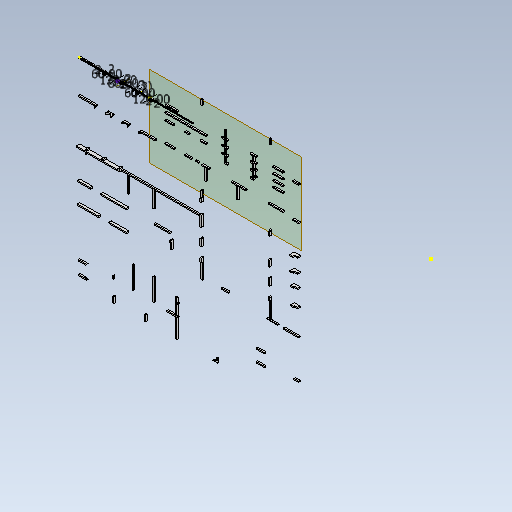
# Autodesk Inventor part: SPRUEs
Saved by Autodesk Inventor 2023 (Build 270158030, 158C)
## iProperties
Created: 2024-12-30
Part Number: SPRUEs
Material: Generic
Document SubType Name: Modeling
Designer: Imogen Heard
Density: 1 g/cm^3
Appearance: Default
Author: Imogen Heard
Autodesk Inventor part; units mm, degrees
(part 1 of 2)
ref_plane "YZ Plane" through (0, 0, 0) normal (1, 0, 0) x (0, 1, 0)
ref_plane "XZ Plane" through (0, 0, 0) normal (0, 1, 0) x (-1, 0, 0)
ref_plane "XY Plane" through (0, 0, 0) normal (0, 0, 1) x (1, 0, 0)
sketch "Sketch1" plane through (0, 0, 0) normal (0, 0, 1) x (1, 0, 0)
  arc A0 (-355.3721, 16.6489) -> (-360.3721, 11.6489) centre (-355.3721, 11.6489) ccw projected
  line L0 (-360.3721, 11.6489) -> (-360.3721, -208.3511) projected
  arc A1 (-360.3721, -208.3511) -> (-355.3721, -213.3511) centre (-355.3721, -208.3511) ccw projected
  line L1 (-355.3721, -213.3511) -> (-135.3721, -213.3511) projected
  arc A2 (-135.3721, -213.3511) -> (-130.3721, -208.3511) centre (-135.3721, -208.3511) ccw projected
  line L2 (-130.3721, -208.3511) -> (-130.3721, 11.6489) projected
  arc A3 (-130.3721, 11.6489) -> (-135.3721, 16.6489) centre (-135.3721, 11.6489) ccw projected
  line L3 (-135.3721, 16.6489) -> (-355.3721, 16.6489) projected
  line L4 (-357.3721, -205.3511) -> (-357.3721, 8.6489) projected
  arc A4 (-352.3721, 13.6489) -> (-357.3721, 8.6489) centre (-352.3721, 8.6489) ccw projected
  line L5 (-352.3721, 13.6489) -> (-138.3721, 13.6489) projected
  arc A5 (-133.3721, 8.6489) -> (-138.3721, 13.6489) centre (-138.3721, 8.6489) ccw projected
  line L6 (-133.3721, 8.6489) -> (-133.3721, -205.3511) projected
  arc A6 (-138.3721, -210.3511) -> (-133.3721, -205.3511) centre (-138.3721, -205.3511) ccw projected
  line L7 (-138.3721, -210.3511) -> (-352.3721, -210.3511) projected
  arc A7 (-357.3721, -205.3511) -> (-352.3721, -210.3511) centre (-352.3721, -205.3511) ccw projected
  line L8 (-139.3721, -46.3511) -> (-139.3721, -11.3511) projected
  arc A8 (-139.3721, -11.3511) -> (-159.3721, 8.6489) centre (-159.3721, -11.3511) ccw projected
  arc A9 (-159.3721, -66.3511) -> (-139.3721, -46.3511) centre (-159.3721, -46.3511) ccw projected
  line L9 (-259.3721, -66.3511) -> (-159.3721, -66.3511) projected
  arc A10 (-279.3721, -46.3511) -> (-259.3721, -66.3511) centre (-259.3721, -46.3511) ccw projected
  line L10 (-279.3721, -11.3511) -> (-279.3721, -46.3511) projected
  arc A11 (-259.3721, 8.6489) -> (-279.3721, -11.3511) centre (-259.3721, -11.3511) ccw projected
  line L11 (-159.3721, 8.6489) -> (-259.3721, 8.6489) projected
  line L12 (-139.3721, -92.3511) -> (-139.3721, -72.8511) projected
  line L13 (-264.3721, -80.2511) -> (-264.3721, -77.8511) projected
  line L14 (-264.3721, -85.8511) -> (-264.3721, -83.4511) projected
  line L15 (-286.3721, 7.6489) -> (-290.1379, 7.6489) projected
  line L16 (-284.3721, -19.3481) -> (-284.3721, 5.6489) projected
  line L17 (-295.1379, 2.6489) -> (-295.1379, -19.3481) projected
  line L18 (-309.4963, -82.3511) -> (-284.3721, -19.3481) projected
  line L19 (-320.2621, -82.3511) -> (-295.1379, -19.3481) projected
  line L20 (-310.5821, -87.3511) -> (-318.1621, -87.3511) projected
  line L21 (-309.4963, -82.3511) -> (-320.2621, -82.3511) projected
  line L22 (-290.1379, 7.6489) -> (-286.3721, 7.6489) projected
  line L23 (-311.9037, -19.3481) -> (-311.9037, 2.6489) projected
  line L24 (-301.1379, -19.3481) -> (-301.1379, 5.6489) projected
  line L25 (-303.1379, 7.6489) -> (-306.9037, 7.6489) projected
  line L26 (-334.9279, -87.3511) -> (-327.3479, -87.3511) projected
  line L27 (-337.0279, -82.3511) -> (-311.9037, -19.3481) projected
  line L28 (-326.2621, -82.3511) -> (-301.1379, -19.3481) projected
  line L29 (-328.6695, 2.6489) -> (-328.6695, -19.3481) projected
  line L30 (-317.9037, 5.6489) -> (-317.9037, -19.3481) projected
  line L31 (-323.6695, 7.6489) -> (-319.9037, 7.6489) projected
  line L32 (-323.6695, 7.6489) -> (-319.9037, 7.6489) projected
  line L33 (-317.9037, -19.3481) -> (-343.0279, -82.3511) projected
  line L34 (-344.1137, -87.3511) -> (-351.6937, -87.3511) projected
  line L35 (-343.0279, -82.3511) -> (-353.7937, -82.3511) projected
  line L36 (-326.2621, -82.3511) -> (-337.0279, -82.3511) projected
  line L37 (-328.6695, -19.3481) -> (-353.7937, -82.3511) projected
  line L38 (-328.6695, -159.3541) -> (-353.7937, -96.3511) projected
  line L39 (-351.6937, -91.3511) -> (-344.1137, -91.3511) projected
  line L40 (-357.3721, -205.3511) -> (-357.3721, 8.6489) projected
  line L41 (-344.3835, -98.3511) -> (-350.843, -98.3511) projected
  line L42 (-353.7937, -96.3511) -> (-343.0279, -96.3511) projected
  line L43 (-343.0279, -96.3511) -> (-317.9037, -159.3541) projected
  line L44 (-344.3835, -80.3511) -> (-350.843, -80.3511) projected
  line L45 (-334.0772, -80.3511) -> (-327.6177, -80.3511) projected
  line L46 (-310.8519, -80.3511) -> (-317.3114, -80.3511) projected
  line L47 (-328.6695, -181.3511) -> (-328.6695, -159.3541) projected
  line L48 (-317.9037, -184.3511) -> (-317.9037, -159.3541) projected
  line L49 (-319.9037, -186.3511) -> (-323.6695, -186.3511) projected
  line L50 (-348.3721, -189.3511) -> (-350.1721, -191.1511) projected
  line L51 (-350.1721, -202.5511) -> (-348.3721, -204.3511) projected
  line L52 (-348.3721, -204.3511) -> (-315.3721, -204.3511) projected
  line L53 (-315.3721, -189.3511) -> (-348.3721, -189.3511) projected
  line L54 (-305.3721, -189.3511) -> (-267.3721, -189.3511) projected
  line L55 (-305.3721, -204.3511) -> (-267.3721, -204.3511) projected
  line L56 (-267.3721, -204.3511) -> (-267.3721, -202.3511) projected
  line L57 (-267.3721, -191.3511) -> (-267.3721, -189.3511) projected
  line L58 (-256.3721, -188.8511) -> (-256.3721, -190.8511) projected
  line L59 (-255.3721, -188.8511) -> (-256.3721, -188.8511) projected
  line L60 (-256.3721, -178.8511) -> (-256.3721, -176.8511) projected
  line L61 (-255.3721, -176.725) -> (-255.3721, -178.8511) projected
  line L62 (-177.3721, -187.8511) -> (-255.3721, -187.8511) projected
  line L63 (-255.3811, -191.985) -> (-220.3631, -196.7172) projected
  line L64 (-177.3631, -191.985) -> (-212.3811, -196.7172) projected
  line L65 (-217.8721, -206.3511) -> (-214.8721, -206.3511) projected
  line L66 (-176.3721, -190.8511) -> (-176.3721, -188.8511) projected
  line L67 (-176.3721, -176.8511) -> (-176.3721, -178.8511) projected
  line L68 (-212.3811, -170.985) -> (-177.3631, -175.7172) projected
  line L69 (-177.3721, -179.8511) -> (-255.3721, -179.8511) projected
  line L70 (-255.3811, -175.7172) -> (-220.3631, -170.985) projected
  line L71 (-217.8721, -161.3511) -> (-214.8721, -161.3511) projected
  line L72 (-168.1757, -199.4489) -> (-168.1757, -171.8085) projected
  line L73 (-139.3555, -200.6287) -> (-166.9959, -200.6287) projected
  line L74 (-138.1757, -171.8085) -> (-138.1757, -199.4489) projected
  line L75 (-166.9959, -170.6287) -> (-139.3555, -170.6287) projected
  spline S0 degree 3 poles (-166.3828, -172.4216) (-166.3184, -172.3571) (-166.2458, -172.3022) (-166.0818, -172.2096) (-165.9909, -172.1749) (-165.7801, -172.1268) (-165.6611, -172.1222) (-165.4156, -172.1541) (-165.2916, -172.1967) (-165.1278, -172.2899) (-165.0777, -172.3249) (-165.0079, -172.3837) (-164.9855, -172.4044) (-164.9474, -172.443) (-164.9314, -172.4605) (-164.8992, -172.498) (-164.8832, -172.5183) (-164.8443, -172.5717) (-164.8224, -172.6057) (-164.7512, -172.7333) (-164.7138, -172.8345) (-164.67, -173.0645) (-164.6692, -173.1941) (-164.7179, -173.4393) (-164.7617, -173.5526) (-164.8861, -173.7526) (-164.9616, -173.8378) (-165.1383, -173.9796) (-165.2367, -174.0339) (-165.449, -174.1095) (-165.5609, -174.1282) (-165.8051, -174.1293) (-165.9347, -174.103) (-166.1122, -174.0306) (-166.1684, -174.0012) (-166.2471, -173.95) (-166.2722, -173.9319) (-166.3151, -173.898) (-166.3332, -173.8826) (-166.3696, -173.8493) (-166.3878, -173.8313) (-166.4323, -173.7838) (-166.4576, -173.7534) (-166.5406, -173.6406) (-166.5883, -173.5503) (-166.6641, -173.3292) (-166.6831, -173.1946) (-166.6644, -172.9351) (-166.6331, -172.8127) (-166.5293, -172.5958) (-166.4637, -172.5025) (-166.3828, -172.4216) knots -0.679682 -0.679682 -0.679682 -0.679682 -0.652333 -0.652333 -0.622445 -0.622445 -0.584314 -0.584314 -0.540491 -0.540491 -0.519433 -0.519433 -0.508858 -0.508858 -0.50064 -0.50064 -0.491726 -0.491726 -0.477797 -0.477797 -0.44161 -0.44161 -0.400083 -0.400083 -0.362912 -0.362912 -0.328842 -0.328842 -0.294828 -0.294828 -0.25925 -0.25925 -0.215821 -0.215821 -0.194179 -0.194179 -0.183492 -0.183492 -0.175261 -0.175261 -0.166401 -0.166401 -0.152709 -0.152709 -0.117956 -0.117956 -0.073549 -0.073549 -0.034305 -0.034305 0 0 0 0 projected
  spline S1 degree 3 poles (-166.3828, -198.8358) (-166.4473, -198.7713) (-166.5022, -198.6988) (-166.5949, -198.5347) (-166.6295, -198.4439) (-166.6776, -198.2331) (-166.6822, -198.1141) (-166.6503, -197.8686) (-166.6078, -197.7446) (-166.5145, -197.5808) (-166.4795, -197.5307) (-166.4207, -197.4609) (-166.4, -197.4385) (-166.3614, -197.4004) (-166.344, -197.3844) (-166.3064, -197.3522) (-166.2862, -197.3362) (-166.2328, -197.2972) (-166.1987, -197.2754) (-166.0711, -197.2042) (-165.9699, -197.1668) (-165.7399, -197.123) (-165.6103, -197.1222) (-165.3651, -197.1709) (-165.2518, -197.2147) (-165.0518, -197.3391) (-164.9666, -197.4146) (-164.8248, -197.5913) (-164.7705, -197.6897) (-164.695, -197.902) (-164.6763, -198.0138) (-164.6751, -198.2581) (-164.7014, -198.3877) (-164.7738, -198.5652) (-164.8032, -198.6214) (-164.8544, -198.7) (-164.8725, -198.7252) (-164.9064, -198.7681) (-164.9219, -198.7862) (-164.9552, -198.8226) (-164.9731, -198.8408) (-165.0206, -198.8852) (-165.051, -198.9106) (-165.1638, -198.9936) (-165.2541, -199.0413) (-165.4752, -199.1171) (-165.6098, -199.136) (-165.8694, -199.1173) (-165.9917, -199.0861) (-166.2087, -198.9823) (-166.302, -198.9167) (-166.3828, -198.8358) knots -0.679682 -0.679682 -0.679682 -0.679682 -0.652333 -0.652333 -0.622445 -0.622445 -0.584314 -0.584314 -0.540491 -0.540491 -0.519433 -0.519433 -0.508858 -0.508858 -0.50064 -0.50064 -0.491726 -0.491726 -0.477797 -0.477797 -0.44161 -0.44161 -0.400083 -0.400083 -0.362912 -0.362912 -0.328842 -0.328842 -0.294828 -0.294828 -0.25925 -0.25925 -0.215821 -0.215821 -0.194179 -0.194179 -0.183492 -0.183492 -0.175261 -0.175261 -0.166401 -0.166401 -0.152709 -0.152709 -0.117956 -0.117956 -0.073549 -0.073549 -0.034305 -0.034305 0 0 0 0 projected
  spline S2 degree 3 poles (-139.9686, -198.8358) (-140.0331, -198.9003) (-140.1056, -198.9552) (-140.2697, -199.0478) (-140.3605, -199.0825) (-140.5713, -199.1306) (-140.6903, -199.1352) (-140.9359, -199.1033) (-141.0598, -199.0607) (-141.2237, -198.9675) (-141.2737, -198.9325) (-141.3435, -198.8737) (-141.3659, -198.853) (-141.404, -198.8144) (-141.42, -198.7969) (-141.4522, -198.7594) (-141.4682, -198.7391) (-141.5072, -198.6857) (-141.529, -198.6517) (-141.6003, -198.5241) (-141.6377, -198.4229) (-141.6815, -198.1929) (-141.6823, -198.0633) (-141.6335, -197.8181) (-141.5897, -197.7048) (-141.4653, -197.5048) (-141.3899, -197.4196) (-141.2131, -197.2778) (-141.1147, -197.2235) (-140.9024, -197.1479) (-140.7906, -197.1292) (-140.5463, -197.1281) (-140.4167, -197.1544) (-140.2392, -197.2268) (-140.183, -197.2562) (-140.1044, -197.3074) (-140.0792, -197.3255) (-140.0363, -197.3594) (-140.0182, -197.3749) (-139.9819, -197.4081) (-139.9637, -197.4261) (-139.9192, -197.4736) (-139.8939, -197.504) (-139.8108, -197.6168) (-139.7632, -197.7071) (-139.6873, -197.9282) (-139.6684, -198.0628) (-139.6871, -198.3223) (-139.7183, -198.4447) (-139.8222, -198.6616) (-139.8878, -198.7549) (-139.9686, -198.8358) knots -0.679682 -0.679682 -0.679682 -0.679682 -0.652333 -0.652333 -0.622445 -0.622445 -0.584314 -0.584314 -0.540491 -0.540491 -0.519433 -0.519433 -0.508858 -0.508858 -0.50064 -0.50064 -0.491726 -0.491726 -0.477797 -0.477797 -0.44161 -0.44161 -0.400083 -0.400083 -0.362912 -0.362912 -0.328842 -0.328842 -0.294828 -0.294828 -0.25925 -0.25925 -0.215821 -0.215821 -0.194179 -0.194179 -0.183492 -0.183492 -0.175261 -0.175261 -0.166401 -0.166401 -0.152709 -0.152709 -0.117956 -0.117956 -0.073549 -0.073549 -0.034305 -0.034305 0 0 0 0 projected
  spline S3 degree 3 poles (-139.9686, -172.4216) (-139.9041, -172.4861) (-139.8492, -172.5586) (-139.7566, -172.7227) (-139.722, -172.8135) (-139.6738, -173.0243) (-139.6692, -173.1433) (-139.7011, -173.3888) (-139.7437, -173.5128) (-139.837, -173.6766) (-139.8719, -173.7267) (-139.9308, -173.7965) (-139.9515, -173.8189) (-139.99, -173.857) (-140.0075, -173.873) (-140.0451, -173.9052) (-140.0653, -173.9212) (-140.1187, -173.9602) (-140.1528, -173.982) (-140.2803, -174.0532) (-140.3815, -174.0906) (-140.6115, -174.1344) (-140.7411, -174.1352) (-140.9864, -174.0865) (-141.0996, -174.0427) (-141.2996, -173.9183) (-141.3848, -173.8428) (-141.5266, -173.6661) (-141.5809, -173.5677) (-141.6565, -173.3554) (-141.6752, -173.2436) (-141.6764, -172.9993) (-141.65, -172.8697) (-141.5777, -172.6922) (-141.5482, -172.636) (-141.497, -172.5574) (-141.4789, -172.5322) (-141.445, -172.4893) (-141.4296, -172.4712) (-141.3963, -172.4348) (-141.3783, -172.4166) (-141.3309, -172.3722) (-141.3004, -172.3468) (-141.1876, -172.2638) (-141.0973, -172.2161) (-140.8762, -172.1403) (-140.7416, -172.1214) (-140.4821, -172.1401) (-140.3597, -172.1713) (-140.1428, -172.2751) (-140.0495, -172.3407) (-139.9686, -172.4216) knots -0.679682 -0.679682 -0.679682 -0.679682 -0.652333 -0.652333 -0.622445 -0.622445 -0.584314 -0.584314 -0.540491 -0.540491 -0.519433 -0.519433 -0.508858 -0.508858 -0.50064 -0.50064 -0.491726 -0.491726 -0.477797 -0.477797 -0.44161 -0.44161 -0.400083 -0.400083 -0.362912 -0.362912 -0.328842 -0.328842 -0.294828 -0.294828 -0.25925 -0.25925 -0.215821 -0.215821 -0.194179 -0.194179 -0.183492 -0.183492 -0.175261 -0.175261 -0.166401 -0.166401 -0.152709 -0.152709 -0.117956 -0.117956 -0.073549 -0.073549 -0.034305 -0.034305 0 0 0 0 projected
  circle A12 centre (-153.1757, -185.6287) radius 3 projected
  spline S4 degree 3 poles (-148.8989, -145.1578) (-148.8663, -145.2434) (-148.839, -145.3309) (-148.7526, -145.6882) (-148.7409, -145.9642) (-148.8289, -146.5268) (-148.9339, -146.8021) (-149.2681, -147.3464) (-149.5104, -147.5979) (-150.1323, -148.0483) (-150.5268, -148.2212) (-151.3838, -148.424) (-151.8499, -148.4418) (-152.6494, -148.3191) (-152.9891, -148.214) (-153.5655, -147.9256) (-153.8098, -147.7577) (-154.2292, -147.356) (-154.4037, -147.1255) (-154.6596, -146.6092) (-154.7368, -146.33) (-154.7716, -145.762) (-154.7323, -145.4845) (-154.5381, -144.9245) (-154.3742, -144.6555) (-153.9118, -144.1374) (-153.5973, -143.9109) (-152.9428, -143.5977) (-152.6093, -143.4993) (-151.9298, -143.4014) (-151.5828, -143.4016) (-150.877, -143.5041) (-150.5185, -143.6147) (-149.8769, -143.9427) (-149.5919, -144.1542) (-149.1611, -144.6332) (-149.0033, -144.8834) (-148.8989, -145.1578) knots -1.730763 -1.730763 -1.730763 -1.730763 -1.703218 -1.703218 -1.620235 -1.620235 -1.532045 -1.532045 -1.428588 -1.428588 -1.3023 -1.3023 -1.165882 -1.165882 -1.060948 -1.060948 -0.972967 -0.972967 -0.886826 -0.886826 -0.800067 -0.800067 -0.716091 -0.716091 -0.622376 -0.622376 -0.508288 -0.508288 -0.40586 -0.40586 -0.303624 -0.303624 -0.193192 -0.193192 -0.088285 -0.088285 0 0 0 0 projected
  arc A13 (-176.8395, -141.8511) -> (-181.3395, -141.8511) centre (-179.0895, -141.8511) ccw projected
  line L76 (-166.0395, -146.5637) -> (-166.0395, -145.5637) projected
  line L77 (-185.6895, -139.6011) -> (-185.6895, -140.8011) projected
  arc A14 (-184.6395, -141.8511) -> (-185.6895, -140.8011) centre (-185.6895, -141.8511) ccw projected
  line L78 (-184.6395, -141.8511) -> (-184.6395, -144.1637) projected
  arc A15 (-184.6395, -144.1637) -> (-180.1395, -144.1637) centre (-182.3895, -144.1637) ccw projected
  line L79 (-180.1395, -144.1637) -> (-180.1395, -141.8511) projected
  arc A16 (-178.0395, -141.8511) -> (-180.1395, -141.8511) centre (-179.0895, -141.8511) ccw projected
  line L80 (-178.0395, -141.8511) -> (-178.0395, -144.1637) projected
  arc A17 (-178.0395, -144.1637) -> (-173.0395, -144.1637) centre (-175.5395, -144.1637) ccw projected
  line L81 (-173.0395, -144.1637) -> (-173.0395, -141.8511) projected
  arc A18 (-170.4395, -141.8511) -> (-173.0395, -141.8511) centre (-171.7395, -141.8511) ccw projected
  line L82 (-170.4395, -141.8511) -> (-170.4395, -144.1637) projected
  arc A19 (-170.4395, -144.1637) -> (-167.6895, -146.6512) centre (-167.9395, -144.1637) ccw projected
  line L83 (-167.6895, -146.6512) -> (-167.6895, -146.5637) projected
  line L84 (-167.6895, -146.5637) -> (-166.0395, -146.5637) projected
  line L85 (-166.0395, -146.5637) -> (-166.0395, -145.5637) projected
  line L86 (-166.0395, -145.5637) -> (-167.6895, -145.5637) projected
  line L87 (-167.6895, -145.5637) -> (-167.6895, -145.4637) projected
  line L88 (-167.6895, -145.4637) -> (-167.9395, -145.4637) projected
  arc A20 (-169.2395, -144.1637) -> (-167.9395, -145.4637) centre (-167.9395, -144.1637) ccw projected
  line L89 (-169.2395, -144.1637) -> (-169.2395, -141.8511) projected
  arc A21 (-169.2395, -141.8511) -> (-174.2395, -141.8511) centre (-171.7395, -141.8511) ccw projected
  line L90 (-174.2395, -141.8511) -> (-174.2395, -144.1637) projected
  arc A22 (-176.8395, -144.1637) -> (-174.2395, -144.1637) centre (-175.5395, -144.1637) ccw projected
  line L91 (-176.8395, -144.1637) -> (-176.8395, -141.8511) projected
  arc A23 (-176.8395, -141.8511) -> (-181.3395, -141.8511) centre (-179.0895, -141.8511) ccw projected
  line L92 (-181.3395, -141.8511) -> (-181.3395, -144.1637) projected
  arc A24 (-183.4395, -144.1637) -> (-181.3395, -144.1637) centre (-182.3895, -144.1637) ccw projected
  line L93 (-183.4395, -144.1637) -> (-183.4395, -141.8511) projected
  arc A25 (-183.4395, -141.8511) -> (-185.6895, -139.6011) centre (-185.6895, -141.8511) ccw projected
  line L94 (-185.6895, -138.1488) -> (-203.7918, -138.1488) projected
  line L95 (-185.6895, -139.6011) -> (-185.6895, -139.0695) projected
  line L96 (-185.6895, -146.9453) -> (-185.6895, -140.8011) projected
  line L97 (-185.6895, -147.866) -> (-203.7918, -147.866) projected
  line L98 (-204.6895, -139.0466) -> (-204.6895, -146.9682) projected
  arc A26 (-237.2273, -141.8432) -> (-240.4148, -141.4877) centre (-239.2273, -145.3073) ccw projected
  arc A27 (-240.4148, -141.4877) -> (-242.7461, -142.5569) centre (-237.446, -151.0368) ccw projected
  arc A28 (-246.8662, -142.6291) -> (-242.7461, -142.5569) centre (-244.8662, -139.165) ccw projected
  line L99 (-246.8662, -142.6291) -> (-262.1246, -133.8196) projected
  arc A29 (-262.1246, -133.8196) -> (-264.146, -134.3227) centre (-262.8746, -135.1187) ccw projected
  arc A30 (-264.146, -134.3227) -> (-264.9229, -135.6332) centre (-237.446, -151.0368) ccw projected
  arc A31 (-264.9229, -135.6332) -> (-265.9735, -137.6789) centre (-265.4669, -136.6465) ccw projected
  arc A32 (-266.8384, -139.708) -> (-265.9735, -137.6789) centre (-267.3412, -138.2948) ccw projected
  arc A33 (-266.8384, -139.708) -> (-268.3318, -140.4513) centre (-267.2323, -140.7884) ccw projected
  arc A34 (-268.3318, -140.4513) -> (-267.6083, -141.9544) centre (-267.2566, -140.8595) ccw projected
  arc A35 (-268.1699, -144.0875) -> (-267.6083, -141.9544) centre (-268.8723, -142.7621) ccw projected
  arc A36 (-268.1699, -144.0875) -> (-269.5398, -145.0394) centre (-268.4031, -145.2136) ccw projected
  arc A37 (-269.5398, -145.0394) -> (-268.6061, -146.4218) centre (-268.4169, -145.2875) ccw projected
  arc A38 (-268.8527, -148.6138) -> (-268.6061, -146.4218) centre (-269.7397, -147.4041) ccw projected
  arc A39 (-268.8527, -148.6138) -> (-270.0702, -149.7542) centre (-268.9202, -149.7618) ccw projected
  arc A40 (-270.0702, -149.7542) -> (-268.946, -150.9866) centre (-268.9232, -149.8368) ccw projected
  arc A41 (-268.8723, -153.1912) -> (-268.946, -150.9866) centre (-269.9253, -152.1229) ccw projected
  arc A42 (-268.8723, -153.1912) -> (-269.9147, -154.4724) centre (-268.7727, -154.3368) ccw projected
  arc A43 (-269.9147, -154.4724) -> (-268.6272, -155.5072) centre (-268.7696, -154.366) ccw projected
  arc A44 (-268.2379, -157.6783) -> (-268.6272, -155.5072) centre (-269.4333, -156.7722) ccw projected
  arc A45 (-268.2379, -157.6783) -> (-269.0857, -159.0959) centre (-267.975, -158.7978) ccw projected
  arc A46 (-269.0857, -159.0959) -> (-267.6631, -159.9352) centre (-267.9678, -158.8263) ccw projected
  arc A47 (-266.9663, -162.028) -> (-267.6631, -159.9352) centre (-268.2793, -161.3027) ccw projected
  arc A48 (-266.9663, -162.028) -> (-267.6019, -163.5525) centre (-266.5454, -163.0982) ccw projected
  arc A49 (-267.6019, -163.5525) -> (-266.0735, -164.179) centre (-266.5342, -163.1253) ccw projected
  arc A50 (-265.0837, -166.1502) -> (-266.0735, -164.179) centre (-266.4871, -165.6209) ccw projected
  arc A51 (-265.0837, -166.1502) -> (-265.4939, -167.7502) centre (-264.5136, -167.1489) ccw projected
  arc A52 (-265.4939, -167.7502) -> (-263.8915, -168.1508) centre (-264.4986, -167.1741) ccw projected
  arc A53 (-262.629, -169.9596) -> (-263.8915, -168.1508) centre (-264.0939, -169.6371) ccw projected
  arc A54 (-262.629, -169.9596) -> (-261.1814, -171.7464) centre (-261.9215, -170.8662) ccw projected
  arc A55 (-261.1814, -171.7464) -> (-259.6868, -173.3437) centre (-237.446, -151.0368) ccw projected
  arc A56 (-259.6868, -173.3437) -> (-257.2844, -173.342) centre (-258.4865, -172.1399) ccw projected
  line L100 (-257.2844, -173.342) -> (-256.8602, -172.9177) projected
  arc A57 (-256.8602, -172.9177) -> (-256.862, -170.5117) centre (-258.0623, -171.7156) ccw projected
  arc A58 (-262.4136, -139.5099) -> (-256.862, -170.5117) centre (-237.446, -151.0368) ccw projected
  line L101 (-262.4136, -139.5099) -> (-239.8503, -152.5368) projected
  arc A59 (-239.8503, -152.5368) -> (-211.7609, -144.125) centre (-230.8896, -131.3542) ccw projected
  arc A60 (-211.7609, -144.125) -> (-214.5101, -142.129) centre (-213.1748, -143.181) ccw projected
  arc A61 (-223.6642, -148.5619) -> (-214.5101, -142.129) centre (-229.8277, -130.0617) ccw projected
  arc A62 (-228.2157, -147.0461) -> (-223.6642, -148.5619) centre (-224.9285, -144.767) ccw projected
  line L102 (-228.2157, -147.0461) -> (-237.2273, -141.8432) projected
  circle A63 centre (-237.446, -151.0368) radius 1 projected
  line L103 (-307.5721, -106.9247) -> (-307.5721, -166.7775) projected
  line L104 (-307.5721, -166.7775) -> (-280.3721, -166.7775) projected
  line L105 (-280.3721, -106.9247) -> (-280.3721, -166.7775) projected
  line L106 (-307.5721, -106.9247) -> (-280.3721, -106.9247) projected
  line L107 (-264.3721, -98.3511) -> (-144.3721, -98.3511) projected
  line L108 (-144.3721, -108.3511) -> (-264.3721, -108.3511) projected
  line L109 (-139.3721, -99.5611) -> (-139.3721, -107.1411) projected
  line L110 (-139.3721, -124.1411) -> (-139.3721, -116.5611) projected
  line L111 (-139.3721, -124.1411) -> (-139.3721, -116.5611) projected
  line L112 (-140.5721, -116.5611) -> (-140.5721, -124.1411) projected
  line L113 (-140.5721, -107.1411) -> (-140.5721, -99.5611) projected
  line L114 (-164.3721, -71.3511) -> (-141.3721, -71.3511) projected
  line L115 (-141.3721, -92.3511) -> (-164.3721, -92.3511) projected
  line L116 (-254.3721, -77.8511) -> (-174.1547, -72.0576) projected
  line L117 (-174.1547, -91.6446) -> (-254.3721, -85.8511) projected
  line L118 (-144.3721, -125.3511) -> (-264.3721, -125.3511) projected
  line L119 (-144.3721, -115.3511) -> (-264.3721, -115.3511) projected
  line L120 (-264.3721, -116.8511) -> (-264.3721, -123.8511) projected
  line L121 (-264.3721, -106.8511) -> (-264.3721, -99.8511) projected
  line L122 (-357.3721, -202.8219) -> (-348.7013, -202.8219)
  line L123 (-348.7013, -202.8219) -> (-348.7013, -204.0219)
  line L124 (-348.7013, -204.0219) -> (-357.3721, -204.0219)
  line L125 (-357.3721, -204.0219) -> (-357.3721, -202.8219)
  line L126 (-348.8045, -203.9187) -> (-350.7013, -203.9187)
  line L127 (-350.7013, -203.9187) -> (-350.7013, -202.9187)
  line L128 (-350.7013, -202.9187) -> (-348.8045, -202.9187)
  line L129 (-348.8045, -202.9187) -> (-348.8045, -203.9187)
  line L130 (-350.7013, -202.8219) -> (-350.7013, -204.0219)
  line L131 (-357.3721, -189.8511) -> (-348.3721, -189.8511)
  line L132 (-348.3721, -189.8511) -> (-348.3721, -191.0511)
  line L133 (-348.3721, -191.0511) -> (-357.3721, -191.0511)
  line L134 (-357.3721, -191.0511) -> (-357.3721, -189.8511)
  line L135 (-322.3695, -210.3511) -> (-321.1695, -210.3511)
  line L136 (-321.1695, -210.3511) -> (-321.1695, -204.3511)
  line L137 (-321.1695, -204.3511) -> (-322.3695, -204.3511)
  line L138 (-322.3695, -204.3511) -> (-322.3695, -210.3511)
  line L139 (-322.3695, -189.3511) -> (-321.7866, -189.3511)
  line L140 (-321.7866, -189.3511) -> (-321.7866, -186.3511)
  line L141 (-321.7866, -186.3511) -> (-322.3695, -186.3511)
  line L142 (-322.3695, -186.3511) -> (-322.3695, -189.3511)
  line L143 (-267.3721, -189.6535) -> (-256.3721, -189.6535)
  line L144 (-256.3721, -189.6535) -> (-256.3721, -190.8535)
  line L145 (-256.3721, -190.8535) -> (-267.3721, -190.8535)
  line L146 (-267.3721, -190.8535) -> (-267.3721, -189.6535)
  line L147 (-258.6883, -173.516) -> (-257.4883, -173.516)
  line L148 (-257.4883, -173.516) -> (-257.4883, -210.3511)
  line L149 (-257.4883, -210.3511) -> (-258.6883, -210.3511)
  line L150 (-258.6883, -210.3511) -> (-258.6883, -173.516)
  line L151 (-257.4883, -178.8511) -> (-256.3721, -178.8511)
  line L152 (-256.3721, -178.8511) -> (-256.3721, -177.8511)
  line L153 (-256.3721, -177.8511) -> (-257.4883, -177.8511)
  line L154 (-257.4883, -177.8511) -> (-257.4883, -178.8511)
  line L155 (-263.5827, -125.3511) -> (-262.3827, -125.3511)
  line L156 (-262.3827, -125.3511) -> (-262.3827, -134.1492)
  line L157 (-262.3827, -134.1492) -> (-263.5827, -134.1492)
  line L158 (-263.5827, -134.1492) -> (-263.5827, -125.3511)
  line L159 (-176.3721, -177.1511) -> (-168.1757, -177.1511)
  line L160 (-168.1757, -177.1511) -> (-168.1757, -178.3511)
  line L161 (-168.1757, -178.3511) -> (-176.3721, -178.3511)
  line L162 (-176.3721, -178.3511) -> (-176.3721, -177.1511)
  line L163 (-176.3721, -189.2511) -> (-168.1757, -189.2511)
  line L164 (-168.1757, -189.2511) -> (-168.1757, -190.4511)
  line L165 (-168.1757, -190.4511) -> (-176.3721, -190.4511)
  line L166 (-176.3721, -190.4511) -> (-176.3721, -189.2511)
  line L167 (-211.8448, -142.1221) -> (-204.6895, -142.1221)
  line L168 (-204.6895, -142.1221) -> (-204.6895, -143.3221)
  line L169 (-204.6895, -143.3221) -> (-211.8448, -143.3221)
  line L170 (-211.8448, -143.3221) -> (-211.8448, -142.1221)
  line L171 (-280.3721, -166.7775) -> (-281.5721, -166.7775)
  line L172 (-281.5721, -166.7775) -> (-281.5721, -189.3511)
  line L173 (-281.5721, -189.3511) -> (-280.3721, -189.3511)
  line L174 (-280.3721, -189.3511) -> (-280.3721, -166.7775)
  line L175 (-307.5721, -106.9247) -> (-307.5721, -166.7775) projected
  line L176 (-307.5721, -166.7775) -> (-280.3721, -166.7775) projected
  line L177 (-280.3721, -106.9247) -> (-280.3721, -166.7775) projected
  line L178 (-307.5721, -106.9247) -> (-280.3721, -106.9247) projected
  line L179 (-301.5721, -166.7775) -> (-302.7721, -166.7775)
  line L180 (-302.7721, -166.7775) -> (-302.7721, -189.3511)
  line L181 (-302.7721, -189.3511) -> (-301.5721, -189.3511)
  line L182 (-301.5721, -189.3511) -> (-301.5721, -166.7775)
  line L183 (-288.9379, -204.3511) -> (-290.1379, -204.3511)
  line L184 (-290.1379, -204.3511) -> (-290.1379, -210.3511)
  line L185 (-290.1379, -210.3511) -> (-288.9379, -210.3511)
  line L186 (-288.9379, -210.3511) -> (-288.9379, -204.3511)
  line L187 (-215.8721, -206.3511) -> (-217.0721, -206.3511)
  line L188 (-217.0721, -206.3511) -> (-217.0721, -210.3511)
  line L189 (-217.0721, -210.3511) -> (-215.8721, -210.3511)
  line L190 (-215.8721, -210.3511) -> (-215.8721, -206.3511)
  line L191 (-166.0395, -146.3637) -> (-154.7094, -146.3637)
  line L192 (-154.7094, -146.3637) -> (-154.7094, -145.7637)
  line L193 (-154.7094, -145.7637) -> (-166.0395, -145.7637)
  line L194 (-166.0395, -145.7637) -> (-166.0395, -146.3637)
  line L195 (-149.8827, -145.7637) -> (-133.3721, -145.7637)
  line L196 (-133.3721, -145.7637) -> (-133.3721, -146.9637)
  line L197 (-133.3721, -146.9637) -> (-149.8827, -146.9637)
  line L198 (-149.8827, -146.9637) -> (-149.8827, -145.7637)
  line L199 (-133.3721, -119.5611) -> (-139.3721, -119.5611)
  line L200 (-139.3721, -119.5611) -> (-139.3721, -120.7611)
  line L201 (-139.3721, -120.7611) -> (-133.3721, -120.7611)
  line L202 (-133.3721, -120.7611) -> (-133.3721, -119.5611)
  line L203 (-133.3721, -102.5611) -> (-139.3721, -102.5611)
  line L204 (-139.3721, -102.5611) -> (-139.3721, -103.7611)
  line L205 (-139.3721, -103.7611) -> (-133.3721, -103.7611)
  line L206 (-133.3721, -103.7611) -> (-133.3721, -102.5611)
  line L207 (-139.3721, -74.8511) -> (-133.3721, -74.8511)
  line L208 (-133.3721, -74.8511) -> (-133.3721, -76.0511)
  line L209 (-133.3721, -76.0511) -> (-139.3721, -76.0511)
  line L210 (-139.3721, -76.0511) -> (-139.3721, -74.8511)
  line L211 (-133.3721, -89.1511) -> (-139.3721, -89.1511)
  line L212 (-139.3721, -89.1511) -> (-139.3721, -90.3511)
  line L213 (-139.3721, -90.3511) -> (-133.3721, -90.3511)
  line L214 (-133.3721, -90.3511) -> (-133.3721, -89.1511)
  line L215 (-231.5215, -66.3511) -> (-232.7215, -66.3511)
  line L216 (-232.7215, -145.1375) -> (-231.5215, -145.1375)
  line L217 (-232.7215, 8.6489) -> (-231.5215, 8.6489)
  line L218 (-231.5215, 8.6489) -> (-231.5215, 13.6489)
  line L219 (-231.5215, 13.6489) -> (-232.7215, 13.6489)
  line L220 (-232.7215, 13.6489) -> (-232.7215, 8.6489)
  line L221 (-232.7215, -66.3511) -> (-232.7215, -76.2874)
  line L222 (-231.5215, -76.2008) -> (-231.5215, -66.3511)
  line L223 (-232.7215, -87.4147) -> (-232.7215, -98.3511)
  line L224 (-231.5215, -98.3511) -> (-231.5215, -87.5014)
  line L225 (-232.7215, -108.3511) -> (-232.7215, -115.3511)
  line L226 (-232.7215, -125.3511) -> (-232.7215, -145.1375)
  line L227 (-231.5215, -145.1375) -> (-231.5215, -125.3511)
  line L228 (-231.5215, -115.3511) -> (-231.5215, -108.3511)
  line L229 (-163.2859, -71.27) -> (-162.0859, -71.27)
  line L230 (-162.0859, 13.6489) -> (-163.2859, 13.6489)
  line L231 (-163.2859, 13.6489) -> (-163.2859, 8.6489)
  line L232 (-163.2859, -66.3511) -> (-163.2859, -71.27)
  line L233 (-162.0859, -71.27) -> (-162.0859, -66.3511)
  line L234 (-162.0859, 8.6489) -> (-162.0859, 13.6489)
  line L235 (-160.3745, -145.7637) -> (-163.2859, -145.7637)
  line L236 (-163.2859, -92.3511) -> (-162.0859, -92.3511)
  line L237 (-162.0859, -145.7637) -> (-163.2859, -145.7637)
  line L238 (-163.2859, -98.3511) -> (-163.2859, -92.3511)
  line L239 (-162.0859, -92.3511) -> (-162.0859, -98.3511)
  line L240 (-163.2859, -98.3511) -> (-163.2859, -92.3511)
  line L241 (-163.2859, -145.7637) -> (-163.2859, -125.3511)
  line L242 (-163.2859, -115.3511) -> (-163.2859, -108.3511)
  line L243 (-162.0859, -108.3511) -> (-162.0859, -115.3511)
  line L244 (-162.0859, -125.3511) -> (-162.0859, -145.7637)
  line L245 (-163.2859, -145.7637) -> (-163.2859, -125.3511)
  line L246 (-163.2859, -115.3511) -> (-163.2859, -108.3511)
  line L247 (-357.3721, -11.3511) -> (-357.3721, -12.5511)
  line L248 (-133.3721, -12.5511) -> (-133.3721, -11.3511)
  line L249 (-133.3721, -11.3511) -> (-139.3721, -11.3511)
  line L250 (-139.3721, -12.5511) -> (-133.3721, -12.5511)
  line L251 (-279.3721, -11.3511) -> (-284.3721, -11.3511)
  line L252 (-284.3721, -12.5511) -> (-279.3721, -12.5511)
  line L253 (-295.1379, -11.3511) -> (-301.1379, -11.3511)
  line L254 (-301.1379, -12.5511) -> (-295.1379, -12.5511)
  line L255 (-311.9037, -11.3511) -> (-317.9037, -11.3511)
  line L256 (-328.6695, -11.3511) -> (-357.3721, -11.3511)
  line L257 (-357.3721, -12.5511) -> (-328.6695, -12.5511)
  line L258 (-317.9037, -12.5511) -> (-311.9037, -12.5511)
  line L259 (-357.3721, -45.1511) -> (-357.3721, -46.3511)
  line L260 (-133.3721, -46.3511) -> (-133.3721, -45.1511)
  line L261 (-133.3721, -45.1511) -> (-139.3721, -45.1511)
  line L262 (-139.3721, -46.3511) -> (-133.3721, -46.3511)
  line L263 (-279.3721, -45.1511) -> (-294.6618, -45.1511)
  line L264 (-295.1403, -46.3511) -> (-279.3721, -46.3511)
  line L265 (-305.4276, -45.1511) -> (-311.4276, -45.1511)
  line L266 (-311.9061, -46.3511) -> (-305.9061, -46.3511)
  line L267 (-322.1934, -45.1511) -> (-328.1934, -45.1511)
  line L268 (-338.9592, -45.1511) -> (-357.3721, -45.1511)
  line L269 (-357.3721, -46.3511) -> (-339.4377, -46.3511)
  line L270 (-328.6719, -46.3511) -> (-322.6719, -46.3511)
  line L271 (-357.3721, -88.7511) -> (-231.5215, -88.7511)
  line L272 (-231.5215, -88.7511) -> (-231.5215, -89.9511)
  line L273 (-231.5215, -89.9511) -> (-357.3721, -89.9511)
  line L274 (-357.3721, -89.9511) -> (-357.3721, -88.7511)
  line L275 (-313.8821, -87.3511) -> (-315.0821, -87.3511)
  line L276 (-315.0821, -87.3511) -> (-315.0821, -88.7511)
  line L277 (-315.0821, -88.7511) -> (-313.8821, -88.7511)
  line L278 (-313.8821, -88.7511) -> (-313.8821, -87.3511)
  line L279 (-330.6479, -87.3511) -> (-331.8479, -87.3511)
  line L280 (-331.8479, -87.3511) -> (-331.8479, -88.7511)
  line L281 (-331.8479, -88.7511) -> (-330.6479, -88.7511)
  line L282 (-330.6479, -88.7511) -> (-330.6479, -87.3511)
  line L283 (-347.4137, -87.3511) -> (-348.6137, -87.3511)
  line L284 (-348.6137, -87.3511) -> (-348.6137, -91.3511)
  line L285 (-348.6137, -91.3511) -> (-347.4137, -91.3511)
  line L286 (-347.4137, -91.3511) -> (-347.4137, -87.3511)
  line L287 (-357.3721, -119.5511) -> (-357.3721, -120.7511)
  line L288 (-264.5154, -120.7511) -> (-264.5154, -119.5511)
  line L289 (-264.5154, -119.5511) -> (-280.3721, -119.5511)
  line L290 (-280.3721, -120.7511) -> (-264.5154, -120.7511)
  line L291 (-307.5721, -119.5511) -> (-333.7763, -119.5511)
  line L292 (-344.5421, -119.5511) -> (-357.3721, -119.5511)
  line L293 (-357.3721, -120.7511) -> (-344.0635, -120.7511)
  line L294 (-333.2977, -120.7511) -> (-307.5721, -120.7511)
  line L295 (-280.3721, -106.9247) -> (-281.5721, -106.9247)
  line L296 (-281.5721, -106.9247) -> (-281.5721, -89.9511)
  line L297 (-281.5721, -89.9511) -> (-280.3721, -89.9511)
  line L298 (-280.3721, -89.9511) -> (-280.3721, -106.9247)
  line L299 (-307.5721, -106.9247) -> (-306.3721, -106.9247)
  line L300 (-306.3721, -106.9247) -> (-306.3721, -89.9511)
  line L301 (-306.3721, -89.9511) -> (-307.5721, -89.9511)
  line L302 (-307.5721, -89.9511) -> (-307.5721, -106.9247)
  line L303 (-133.3721, -184.9119) -> (-150.2149, -184.9119)
  line L304 (-150.2149, -184.9119) -> (-150.2149, -186.1119)
  line L305 (-150.2149, -186.1119) -> (-133.3721, -186.1119)
  line L306 (-133.3721, -186.1119) -> (-133.3721, -184.9119)
  line L307 (-357.3721, -140.4513) -> (-357.3721, -141.6513)
  line L308 (-307.5721, -141.6513) -> (-307.5721, -140.4513)
  line L309 (-307.5721, -140.4513) -> (-325.4417, -140.4513)
  line L310 (-336.2075, -140.4513) -> (-357.3721, -140.4513)
  line L311 (-357.3721, -141.6513) -> (-335.729, -141.6513)
  line L312 (-324.9632, -141.6513) -> (-307.5721, -141.6513)
  point P0 (0, 0)
  point P1 (-166.3828, -172.4216)
  point P2 (-166.3828, -198.8358)
  point P3 (-139.9686, -198.8358)
  point P4 (-139.9686, -172.4216)
  point P5 (-208.2672, -142.1221)
  point P6 (-288.9379, -207.3511)
  point P7 (-162.0859, 11.1489)
  point P8 (-347.4137, -88.7511)
  point P9 (-348.6137, -88.7511)
  point P10 (-348.6137, -89.9511)
  point P11 (-347.4137, -89.9511)
  point P12 (-232.7215, -89.9511)
  point P13 (-232.7215, -88.7511)
  point P14 (-350.0721, -191.0511)
  point P15 (-348.8721, -189.8511)
  point P16 (-349.8045, -202.9187)
  point P17 (-258.6883, -189.6535)
  point P18 (-258.6883, -190.8535)
  point P19 (-257.4883, -190.8535)
  point P20 (-257.4883, -189.6535)
  point P21 (-138.1757, -186.1119)
  point P22 (-138.1757, -184.9119)
  point P23 (-150.2149, -185.1455)
  point P24 (-149.0358, -146.9637)
  point P25 (-148.7638, -145.7637)
  point P26 (-211.4806, -143.3221)
  point P27 (-263.5827, -133.7963)
  point P28 (-262.3827, -133.7016)
  point P29 (-232.7215, -144.4446)
  dimension "d0" = 1.2
  dimension "d1" = 0.3292
  dimension "d2" = 1
  dimension "d3" = 0.1032
  dimension "d4" = 2
  dimension "d5" = 1.2
  dimension "d6" = 0.5
  dimension "d7" = 1.2
  dimension "d8" = 1.3
  dimension "d9" = 1.2
  dimension "d10" = 0.3024
  dimension "d11" = 1.2
  dimension "d13" = 1
  dimension "d14" = 1.2
  dimension "d15" = 1.3402
  dimension "d16" = 1.1162
  dimension "d17" = 1.2
  dimension "d18" = 1.2
  dimension "d19" = 1.4339
  dimension "d20" = 1.4
  dimension "d21" = 3.9733
  dimension "d22" = 1.2
  dimension "d23" = 1.2
  dimension "d24" = 1.2
  dimension "d25" = 20
  dimension "d26" = 1.2
  dimension "d27" = 21.5658
  dimension "d28" = 1.2
  dimension "d29" = 1
  dimension "d30" = 0.6
  dimension "d31" = 0.2
  dimension "d32" = 1.2
  dimension "d33" = 16.5106
  dimension "d34" = 1.2
  dimension "d35" = 3
  dimension "d36" = 3
  dimension "d37" = 1.2
  dimension "d38" = 1.2
  dimension "d39" = 2
  dimension "d40" = 2
  dimension "d41" = 1.2
  dimension "d43" = 1.2
  dimension "d44" = 46.6506
  dimension "d46" = 1.2
  dimension "d47" = 22.7138
  dimension "d49" = 1.2
  dimension "d51" = 1.2
  dimension "d52" = 1.2
  dimension "d53" = 1.4
  dimension "d54" = 1.4
  dimension "d55" = 1.2
  dimension "d56" = 1.2
  dimension "d57" = 1.2
  dimension "d58" = 3.3
  dimension "d59" = 3.3
  dimension "d60" = 3.3
  dimension "d63" = 4.2
  dimension "d64" = 1.2
  dimension "d65" = 1.2
  dimension "d66" = 1.2
  dimension "d67" = 1.2
  dimension "d68" = 14.5168
  dimension "d69" = 1.2
  dimension "d70" = 20.9002
  constraints: 375 end point, 159 parallel, 110 point on line, 55 perpendicular, 48 horizontal, 23 horizontal alignment, 20 vertical alignment, 6 midpoint, 5 point on circle, 1 coincident, 21 other
  measures "d0" distance between parallel lines of L124 L122
  measures "d1" distance between parallel lines of L52 L124
  measures "d2" distance between parallel lines of L126 L128
  measures "d3" distance between parallel lines of L126 L124
  measures "d4" distance between parallel lines of L123 L127
  measures "d5" distance between parallel lines of L133 L131
  measures "d6" distance between parallel lines of L53 L131
  measures "d7" distance between parallel lines of L136 L138
  measures "d8" distance from line of L138 L49.end
  measures "d9" distance between parallel lines of L145 L143
  measures "d10" distance between parallel lines of L143 L54
  measures "d11" distance between parallel lines of L150 L148
  measures "d13" distance between parallel lines of L151 L153
  measures "d14" distance between parallel lines of L156 L158
  measures "d15" distance from line of L158 A30.end
  measures "d16" distance between parallel lines of L60 L148
  measures "d17" distance between parallel lines of L161 L159
  measures "d18" distance between parallel lines of L165 L163
  measures "d19" vertical distance of L68.end L159.start
  measures "d20" distance from line of L62 L163.start
  measures "d21" distance from line of point (-208.267, -142.122) L94
  measures "d22" distance between parallel lines of L169 L167
  measures "d23" distance between parallel lines of L172 L174
  measures "d24" distance between parallel lines of L180 L182
  measures "d25" distance between parallel lines of L172 L182
  measures "d26" distance from line of L184 point (-288.938, -207.351)
  measures "d27" distance from line of L55.end L186
  measures "d28" distance between parallel lines of L188 L190
  measures "d29" distance from line of L65.end L190
  measures "d30" distance between parallel lines of L191 L193
  measures "d31" distance between parallel lines of L86 L193
  measures "d32" distance between parallel lines of L197 L195
  measures "d33" distance from line of L198 L195.end
  measures "d34" distance between parallel lines of L205 L203
  measures "d35" distance from line of L109.start L203
  measures "d36" distance from line of L199 L110.end
  measures "d37" distance between parallel lines of L201 L199
  measures "d38" distance between parallel lines of L209 L207
  measures "d39" distance from line of L207 L12.end
  measures "d40" distance from line of L213 L12.start
  measures "d41" distance between parallel lines of L213 L211
  measures "d43" distance from line of L218 L217.start
  measures "d44" distance between parallel lines of L10 L220
  measures "d46" distance from line of L231 point (-162.086, 11.149)
  measures "d47" distance between parallel lines of L234 L8
  measures "d49" distance between parallel lines of L250 L249
  measures "d51" distance between parallel lines of L261 L262
  measures "d52" distance between parallel lines of L273 L271
  measures "d53" distance between parallel lines of L34 L271
  measures "d54" distance between parallel lines of L39 L273
  measures "d55" distance between parallel lines of L284 L286
  measures "d56" distance between parallel lines of L280 L282
  measures "d57" distance between parallel lines of L276 L278
  measures "d58" distance from line of L26.end L282
  measures "d59" distance from line of L20.start L278
  measures "d60" distance from line of L34.start L286
  measures "d63" distance between parallel lines of L119 L289
  measures "d64" distance between parallel lines of L290 L289
  measures "d65" distance between parallel lines of L296 L298
  measures "d66" distance between parallel lines of L302 L300
  measures "d67" distance between parallel lines of L303 L305
  measures "d68" distance between parallel lines of L305 L73
  measures "d69" distance between parallel lines of L312 L309
  measures "d70" distance between parallel lines of L291 L309
extrude "Extrusion1" add sketch "Sketch1" along normal blind 1.5 contours L4 L122 L130 L127 L124 | L142 L49 L140 L53 | L138 L52 L136 L7 | L4 L131 L50 L133 | L127 L128 L51 L126 | L184 L55 L186 L7 | L4 L310 L38 L311 | L150 L145 L148 L7 | L4 L292 L38 L293 | L150 L143 L148 L145 | L145 L57 L143 L150 | L188 L65 L190 L7 | L148 L143 L58 L144 L145 | L150 A56 L148 L143 | L238 L115 L239 L107 | L4 L271 L284 L273 | L150 L147 A56 | L284 L271 L286 L273 | L273 L286 L39 L284 | L148 L153 L60 L151 | L4 L268 L37 L269 | L284 L34 L286 L271 | L286 L271 L223 L273 | L54 L172 L104 L174 | L273 L300 L106 L302 | L291 L103 L294 L43 | L305 L74 L303 L6 | L4 L256 L29 L257 | L280 L26 L282 L271 | L54 L180 L104 L182 | L105 L289 L288 L290 | L273 L298 L106 L296 | L309 L103 L312 L43 | L197 S4 L195 L6 | L33 L267 L27 L270 | L276 L20 L278 L271 | L273 L224 L107 L223 | L223 L271 L224 L273 | L201 L110 L199 L6 | L191 L76 L193 S4 | S4 L193 L192 | L5 L218 L11 L220 | L223 L117 L224 L271 | A60 L167 L98 L169 | L30 L255 L23 L258 | L205 L109 L203 L6 | L5 L234 L11 L231 | L28 L265 L19 L266 | L193 L241 L118 L244 | L10 L252 L16 L251 | L213 L12 L211 L6 | L227 L102 L226 L118 | L10 L264 L18 L263 | L24 L253 L17 L254 | L209 L12 L207 L6 | L6 L250 L8 L249 | L156 A29 L158 L118 | L262 L8 L261 L6 | L9 L222 L116 L221 | L9 L233 L229 L232 | L161 L67 L159 L72 | L66 L163 L72 L165 | L243 L119 L242 L108 | L228 L119 L225 L108
ref_plane "Work Plane1" through (-209.3721, -28.8511, 0) normal (0, 0, -1) x (-1, 0, 0)